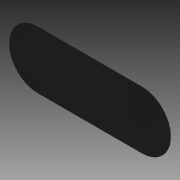
# Autodesk Inventor part: Start_Velostat
Saved by Autodesk Inventor 2014 SP1 (Build 180222100, 222)
## iProperties
Created: 2014-01-13
Part Number: Start_Velostat
Material: Rubber
Document SubType Name: Modeling
Designer: tuleu
Density: 0.93 g/cm^3
Appearance: Rubber - Black - Version 1.1
Author: tuleu
Autodesk Inventor part; units mm, degrees
ref_plane "YZ Plane" through (0, 0, 0) normal (1, 0, 0) x (0, 1, 0)
ref_plane "XZ Plane" through (0, 0, 0) normal (0, 1, 0) x (-1, 0, 0)
ref_plane "XY Plane" through (0, 0, 0) normal (0, 0, 1) x (1, 0, 0)
sketch "Sketch1" plane through (0, 0, 0) normal (0, 1, 0) x (-1, 0, 0)
  line L0 (45, 25) -> (-45, 25)
  line L1 (-45, -25) -> (45, -25)
  arc A0 (-45, 25) -> (-45, -25) centre (-45, 0) ccw
  arc A1 (45, -25) -> (45, 25) centre (45, 0) ccw
  line L2 (45, 0) -> (-45, 0)
  line L3 (0, -25) -> (0, 25)
  point P0 (0, 0)
  dimension "d0" = 90
  dimension "d1" = 50
  constraints: 8 end point, 4 midpoint, 4 point on circle, 3 tangent, 2 centre point, 2 parallel, 1 horizontal
  measures "d0" distance of L2.end L2.start
  measures "d1" distance between parallel lines of L0 L1
extrude "Extrusion1" add sketch "Sketch1" along normal mid plane 0.01
body "Solid1"
